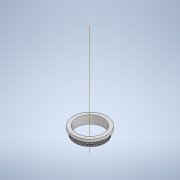
# Autodesk Inventor part: 2020-simulatedFilterWithThread
Saved by Autodesk Inventor 2020.2 (Build 242310000, 310)
## iProperties
Created: 2020-04-14
Part Number: 2020-simulatedFilterWithThread
Material: Generic
Document SubType Name: Modeling
Designer: robst
Density: 1 g/cm^3
Appearance: Default
Author: robst
Autodesk Inventor part; units mm, degrees
ref_plane "YZ Plane" through (0, 0, 0) normal (1, 0, 0) x (0, 1, 0)
ref_plane "XZ Plane" through (0, 0, 0) normal (0, 1, 0) x (-1, 0, 0)
ref_plane "XY Plane" through (0, 0, 0) normal (0, 0, 1) x (1, 0, 0)
sketch "Sketch1" plane through (0, 0, 0) normal (0, 0, 1) x (1, 0, 0)
  line L0 (14.2875, 0) -> (14.2875, 5.08)
  line L1 (14.2875, 5.08) -> (15.875, 5.08)
  line L2 (12.7, 7.62) -> (12.7, 0)
  line L3 (12.7, 0) -> (14.2875, 0)
  line L4 (0, -2.54) -> (0, 15.24) projected
  line L5 (14.2875, 12.7) -> (14.2875, 7.62)
  line L6 (14.2875, 7.62) -> (15.875, 7.62)
  line L7 (15.875, 7.62) -> (15.875, 5.08)
  line L8 (15.875, 7.62) -> (15.875, 12.7)
  line L9 (15.875, 12.7) -> (14.2875, 12.7)
  line L10 (12.7, 7.62) -> (14.2875, 7.62)
  point P0 (0, 0)
  dimension "d1" = 14.2875
  dimension "d2" = 12.7
  dimension "d3" = 5.08
  constraints: 20 end point, 5 perpendicular, 3 vertical, 2 point on line, 1 horizontal
  measures "d1" distance from line of point (0, 0) L0
  measures "d2" distance from line of point (0, 0) L2
  measures "d3" distance of L0.end L0.start
revolve "Revolution1" add sketch "Sketch1" angle 360 about axis through (0, -10, 0) along (0, 1, 0) contours L3 L2 L10 L6 L7 L1 L0
thread "Thread3" size "1 1/8-42 Filter" class "3A" standard "ANSI Unified Screw Threads" full length
sketch "Sketch6" plane through (0, 0, 0) normal (-1, 0, 0) x (0, 0, 1)
  line L0 (14.2875, 0) -> (14.2875, 5.08)
  line L1 (14.2875, 5.08) -> (13.8391, 5.08)
  line L2 (13.8391, 5.08) -> (13.8391, 0)
  line L3 (13.8391, 0) -> (14.2875, 0)
  line L4 (0, -1.016) -> (0, 6.096) projected
  constraints: 8 end point
revolve "Revolution4" cut sketch "Sketch6" angle 360 about axis through (0, 0, 0) along (0, 1, 0)
sketch "Sketch7" plane through (0, 0, 0) normal (-1, 0, 0) x (0, 0, 1)
  line L0 (14.2875, 0) -> (14.2875, 5.08)
  line L1 (14.2875, 5.08) -> (13.8391, 5.08)
  line L2 (13.8391, 5.08) -> (13.8391, 0)
  line L3 (13.8391, 0) -> (14.2875, 0)
  line L4 (0, -1.016) -> (0, 6.096) projected
  constraints: 8 end point
revolve "Revolution5" add sketch "Sketch7" angle 360 about axis through (0, 0, 0) along (0, 1, 0) separate body
sketch "Sketch5" plane through (0, 0, 0) normal (1, 0, 0) x (0, 1, 0)
  line L0 (-0.3529, -13.8698) -> (-0.3025, -13.8698) construction
  line L1 (0.0503, -14.2571) -> (-0.0001, -14.3539) construction
  line L2 (-0.6049, -14.3539) -> (-0.6553, -14.2571) construction
  line L3 (-0.2521, -13.8698) -> (-0.3025, -13.773) construction
  line L4 (-0.3025, -13.773) -> (-0.3529, -13.8698) construction
  line L5 (-0.6049, -14.3539) -> (-0.5545, -14.2571) construction
  line L6 (-0.2521, -13.8698) -> (-0.0505, -14.2571)
  line L7 (-0.6553, -14.2571) -> (-0.5545, -14.2571) construction
  arc A0 (-0.6553, -14.2571) -> (-0.6049, -14.2877) centre (-0.6049, -14.2309) ccw construction
  line L8 (0.0503, -14.2571) -> (-0.0505, -14.2571) construction
  line L9 (-0.6049, -14.3539) -> (-0.6049, -14.2571) construction
  line L10 (-0.0001, -14.3539) -> (-0.0001, -14.2571) construction
  line L11 (-0.3025, -13.773) -> (-0.3025, -13.8393) construction
  line L12 (-0.6049, -14.2877) -> (-0.0001, -14.2877)
  arc A1 (-0.6049, -14.2877) -> (-0.5545, -14.2571) centre (-0.6049, -14.2309) ccw
  line L13 (-0.0505, -14.2571) -> (-0.0001, -14.3539) construction
  line L14 (-0.5545, -14.2571) -> (-0.3529, -13.8698)
  line L15 (-0.0001, -0.0002) -> (-0.0001, 0.0177)
  line L16 (-0.0001, 0.0177) -> (-0.0001, -0.0002)
  line L17 (-0.0001, -0.0002) -> (0.0334, -0.0002)
  arc A2 (-0.0505, -14.2571) -> (-0.0001, -14.2877) centre (-0.0001, -14.2309) ccw
  arc A3 (-0.0001, -14.2877) -> (0.0503, -14.2571) centre (-0.0001, -14.2309) ccw construction
  arc A4 (-0.3025, -13.8393) -> (-0.3529, -13.8698) centre (-0.3025, -13.8961) ccw
  arc A5 (-0.2521, -13.8698) -> (-0.3025, -13.8393) centre (-0.3025, -13.8961) ccw
  line L18 (-0.3025, -13.8393) -> (-0.3025, -13.8698) construction
  line L19 (-0.3025, -13.8698) -> (-0.2521, -13.8698) construction
  dimension "d31" = 55
  dimension "d32" = 0.0968
  dimension "d33" = 0.0968
  dimension "Sketch5_ThreadOffset" = 0
  dimension "Sketch5_MajorRadius" = 14.2875
  dimension "d36" = 0.6048
  dimension "Sketch5_MinorRadius" = 13.8391
  constraints: 40 end point, 12 point on circle, 10 parallel, 8 tangent, 6 centre point, 6 collinear, 2 midpoint, 2 point on line, 1 horizontal, 1 perpendicular, 3 other
  measures "d31" angle of L6 L14
  measures "d32" distance of L3.end L0.end
  measures "d33" distance of L1.end L10.end
  measures "Sketch5_ThreadOffset" distance between parallel lines of L15 L10
  measures "Sketch5_MajorRadius" distance from line of L12 L15.start
  measures "d36" distance from line of L1.end L9
  measures "Sketch5_MinorRadius" distance edge to line of A5 L17
coil "Coil2" sketch "Sketch5" operation cut axis through (0, 0, 0) along (0, 1, 0) pitch 0.6054 turns 10.38961 hand right bodies 2
equation "\"d31\" = d38"
equation "\"d32\" = 0.160083 * Sketch5_Pitch"
equation "\"d33\" = 0.160083 * Sketch5_Pitch"
equation "\"d36\" = Sketch5_Pitch"
equation "\"d15\" = 55deg"
equation "\"Sketch2_Pitch\" = 0.90714"
equation "\"d38\" = 55deg"
equation "\"Sketch5_Pitch\" = 0.60476"
body "Solid1"
body "Solid3"
